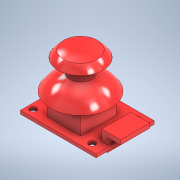
# Autodesk Inventor part: Joystick
Saved by Autodesk Inventor 2020 (Build 240168000, 168)
## iProperties
Created: 2020-01-01
Part Number: Joystick
Material: Argent
Document SubType Name: Modeling
Designer: Manuel Enzo
Density: 10.49 g/cm^3
Appearance: Rouge clair
Author: Manuel Enzo
Autodesk Inventor part; units mm, degrees
ref_plane "YZ Plane" through (0, 0, 0) normal (1, 0, 0) x (0, 1, 0)
ref_plane "XZ Plane" through (0, 0, 0) normal (0, 1, 0) x (-1, 0, 0)
ref_plane "XY Plane" through (0, 0, 0) normal (0, 0, 1) x (1, 0, 0)
sketch "Esquisse1" plane through (0, 0, 0) normal (0, 1, 0) x (-1, 0, 0)
  line L0 (0, 0) -> (34, 0)
  line L1 (34, 0) -> (34, -26)
  line L2 (34, -26) -> (0, -26)
  line L3 (0, -26) -> (0, 0)
  circle A0 centre (31.5, -22.75) radius 2
  circle A1 centre (31.5, -22.75) radius 1.5
  circle A2 centre (31.5, -3.25) radius 2
  circle A3 centre (31.5, -3.25) radius 1.5
  circle A4 centre (5, -3.25) radius 2
  circle A5 centre (5, -3.25) radius 1.5
  circle A6 centre (5, -22.75) radius 2
  circle A7 centre (5, -22.75) radius 1.5
  line L4 (25.5, -3.5) -> (10.5, -3.5)
  line L5 (10.5, -3.5) -> (10.5, -19.5)
  line L6 (10.5, -19.5) -> (25.5, -19.5)
  line L7 (25.5, -19.5) -> (25.5, -3.5)
  line L8 (3.5, -6) -> (1, -6)
  line L9 (1, -6) -> (1, -19)
  line L10 (1, -19) -> (3.5, -19)
  line L11 (3.5, -19) -> (3.5, -6)
  dimension "d0" = 26
  dimension "d1" = 34
  dimension "d2" = 0.5
  dimension "d3" = 4
  dimension "d4" = 2.5
  dimension "d5" = 3.25
  dimension "d6" = 0.5
  dimension "d7" = 4
  dimension "d8" = 2.5
  dimension "d9" = 3.25
  dimension "d10" = 0.5
  dimension "d11" = 0.5
  dimension "d12" = 4
  dimension "d13" = 0.5
  dimension "d14" = 4
  dimension "d15" = 3.25
  dimension "d16" = 3.25
  dimension "d17" = 5
  dimension "d18" = 5
  dimension "d19" = 15
  dimension "d20" = 16
  dimension "d21" = 8.5
  dimension "d22" = 6.5
  dimension "d23" = 3.5
  dimension "d24" = 10.5
  dimension "d25" = 1
  dimension "d26" = 2.5
  dimension "d27" = 7
  dimension "d28" = 6
  constraints: 24 end point, 8 centre point, 6 parallel, 4 coincident, 3 horizontal, 3 perpendicular
  measures "d0" distance between parallel lines of L2 L0
  measures "d1" distance between parallel lines of L3 L1
  measures "d2" radial gap between concentric circles of A0 A1
  measures "d3" diameter of A0
  measures "d4" distance from line of L1 A0.centre
  measures "d5" distance from line of L2 A0.centre
  measures "d6" radial gap between concentric circles of A2 A3
  measures "d7" diameter of A2
  measures "d8" distance from line of L1 A2.centre
  measures "d9" distance from line of L0 A2.centre
  measures "d10" radial gap between concentric circles of A6 A7
  measures "d11" radial gap between concentric circles of A4 A5
  measures "d12" diameter of A4
  measures "d13" radial gap between concentric circles of A6 A7
  measures "d14" diameter of A6
  measures "d15" distance from line of L0 A4.centre
  measures "d16" distance from line of L2 A6.centre
  measures "d17" distance from line of L3 A6.centre
  measures "d18" distance from line of L3 A5.centre
  measures "d19" distance between parallel lines of L7 L5
  measures "d20" distance between parallel lines of L4 L6
  measures "d21" distance between parallel lines of L1 L7
  measures "d22" distance between parallel lines of L2 L6
  measures "d23" distance between parallel lines of L0 L4
  measures "d24" distance between parallel lines of L3 L5
  measures "d25" distance between parallel lines of L3 L9
  measures "d26" distance between parallel lines of L11 L9
  measures "d27" distance between parallel lines of L2 L10
  measures "d28" distance between parallel lines of L0 L8
extrude "Extrusion1" add sketch "Esquisse1" along normal blind 1.5 contours L0 L1 L2 L3 | A0 | A2 | A4 | A6
extrude "Extrusion2" add sketch "Esquisse1" along normal blind 11.5 contours L7 L6 L5 L4
extrude "Extrusion3" add sketch "Esquisse1" along normal blind 6.5 contours L11 L10 L9 L8
sketch "Esquisse2" plane through (0, 11.5, 0) normal (0, 1, 0) x (1, 0, 0)
  line L0 (-10.5, 3.5) -> (-10.5, 19.5) projected
  line L1 (-25.5, 3.5) -> (-25.5, 19.5) projected
  line L2 (-10.5, 11) -> (-25.5, 11)
  line L3 (-25.5, 11) -> (-25.5, 12)
  line L4 (-25.5, 12) -> (-10.5, 12)
  line L5 (-10.5, 12) -> (-10.5, 11)
  line L6 (-25.5, 3.5) -> (-10.5, 3.5) projected
  point P0 (0, 0)
  dimension "d35" = 7.5
  dimension "d36" = 1
  constraints: 8 end point, 2 parallel, 2 point on line, 1 horizontal, 1 perpendicular
  measures "d35" distance between parallel lines of L6 L2
  measures "d36" distance between parallel lines of L2 L4
extrude "Extrusion4" add sketch "Esquisse2" along normal blind 5 contours L2 L1 L4 L0
sketch "Esquisse3" plane through (-25.5, 11.5, -11) normal (0, 0, 1) x (1, 0, 0)
  line L0 (0, 0) -> (15, 0) projected
  line L1 (0, 0) -> (7.5, 0)
  line L2 (0, 0) -> (0, 5) projected
  line L3 (7.5, 0) -> (-6, 0)
  line L4 (7.5, 0) -> (7.5, 7)
  line L5 (7.5, 0) -> (7.5, -14.7162)
  line L6 (0, -10) -> (0, 0) projected
  line L7 (0, 0) -> (0, 5.9)
  arc A0 (2.5, 7) -> (-6, 0) centre (7.4788, -7.7064) ccw
  line L8 (2.5, 7) -> (2.5, 13)
  line L9 (7.5, 13) -> (7.5, 7)
  line L10 (7.5, 13) -> (7.5, 17)
  line L11 (2.5, 13) -> (-2.5, 13)
  line L12 (-8.5, -11.5) -> (25.5, -11.5) projected
  arc A1 (7.5, 17) -> (-0.0106, 15.9926) centre (7.5, -11.5) ccw
  arc A2 (-0.0106, 15.9926) -> (-2.5468, 13.0281) centre (7.5, 7) ccw
  line L13 (-2.5468, 13.0281) -> (-2.5, 13)
  point P0 (2.5, 7)
  dimension "d39" = 7.5
  dimension "d40" = 13.5
  dimension "d41" = 7
  dimension "d42" = 5
  dimension "d43" = 5.9
  dimension "d44" = 5
  dimension "d46" = 4
  dimension "d47" = 5
  constraints: 20 end point, 7 point on circle, 4 vertical, 3 centre point, 2 horizontal, 2 point on line, 1 coincident, 1 midpoint, 1 parallel
  measures "d39" distance from line of L2 L1.end
  measures "d40" distance of L1.end L3.end
  measures "d41" distance of L1.end L4.end
  measures "d42" distance of L4.end A0.start
  measures "d43" distance of L0.start L7.end
  measures "d44" distance between parallel lines of L8 L9
  measures "d46" distance of L9.start L10.end
  measures "d47" distance of L8.end L11.end
revolve "Révolution1" add sketch "Esquisse3" angle 360 about axis through (-18, 24.5, -11) along (0, -1, 0)
sketch "Esquisse4" plane through (-1, 1.5, -19) normal (1, 0, 0) x (0, 0, -1)
  line L0 (0, 5) -> (-13, 5) projected
  line L1 (0, 0) -> (0, 5) projected
  line L2 (-13, 5) -> (0, 5)
  line L3 (0, 5) -> (0, 3)
  line L4 (0, 3) -> (-13, 3)
  line L5 (-13, 3) -> (-13, 5)
  point P0 (-19, -1.5)
  dimension "d50" = 2
  constraints: 8 end point, 2 parallel, 1 horizontal, 1 perpendicular, 1 point on line
  measures "d50" distance between parallel lines of L0 L4
extrude "Extrusion5" add sketch "Esquisse4" along normal blind 6
extrude "Extrusion6" add sketch "Esquisse1" against normal blind 1.5 contours L11 L10 L9 L8
extrude "Extrusion7" add sketch "Esquisse1" against normal blind 2 contours L7 L6 L5 L4
